Autodesk Inventor part; units mm, degrees
(part 2 of 2)
  spline S148 degree 2 poles (-17.7815, 46.7577) (-17.6758, 46.9585) (-17.3312, 47.2573) (-17.0296, 47.3658) knots 0 0 0 1 2 2 2
  spline S149 degree 2 poles (-19.8158, 45.9019) (-19.7815, 45.9593) (-19.669, 46.1603) (-19.607, 46.2324) knots 0 0 0 1 2 2 2
  spline S150 degree 2 poles (-19.607, 46.2324) (-19.5238, 46.335) (-19.3477, 46.4796) (-19.1646, 46.5564) knots 0 0 0 1 2 2 2
  spline S151 degree 2 poles (-19.1646, 46.5564) (-19.0155, 46.6189) (-18.6989, 46.6194) (-18.5541, 46.5602) knots 0 0 0 1 2 2 2
  spline S152 degree 2 poles (-18.5541, 46.5602) (-18.4157, 46.5014) (-18.1751, 46.2578) (-18.1071, 46.0957) knots 0 0 0 1 2 2 2
  spline S153 degree 2 poles (-18.1071, 46.0957) (-18.0018, 45.8446) (-18.0645, 45.4) (-18.2518, 45.2014) knots 0 0 0 1 2 2 2
  spline S154 degree 2 poles (-18.2518, 45.2014) (-18.4164, 45.0217) (-18.9413, 44.7185) (-19.2553, 44.5653) knots 0 0 0 1 2 2 2
  line L139 (-19.2553, 44.5653) -> (-19.2224, 44.4868)
  spline S155 degree 2 poles (-19.2224, 44.4868) (-19.1631, 44.3456) (-19.0033, 44.2065) (-18.904, 44.1898) knots 0 0 0 1 2 2 2
  spline S156 degree 2 poles (-18.904, 44.1898) (-18.8047, 44.173) (-18.5666, 44.2359) (-18.4463, 44.2864) knots 0 0 0 1 2 2 2
  spline S157 degree 2 poles (-18.4463, 44.2864) (-18.305, 44.3456) (-17.9583, 44.5895) (-17.8013, 44.7506) knots 0 0 0 1 2 2 2
  line L140 (-17.8013, 44.7506) -> (-17.7778, 44.7605)
  line L141 (-17.7778, 44.7605) -> (-17.6034, 44.3446)
  spline S158 degree 2 poles (-17.6034, 44.3446) (-17.7027, 44.2661) (-18.0909, 44.011) (-18.2975, 43.9243) knots 0 0 0 1 2 2 2
  spline S159 degree 2 poles (-18.2975, 43.9243) (-18.5486, 43.819) (-18.9242, 43.7538) (-19.103, 43.7988) knots 0 0 0 1 2 2 2
  spline S160 degree 2 poles (-19.103, 43.7988) (-19.278, 43.8422) (-19.5416, 44.1038) (-19.637, 44.3314) knots 0 0 0 1 2 2 2
  line L142 (-19.637, 44.3314) -> (-20.3314, 45.9871)
  line L143 (-20.3314, 45.9871) -> (-19.9234, 46.1582)
  line L144 (-19.9234, 46.1582) -> (-19.8158, 45.9019)
  line L145 (-19.6732, 45.5618) -> (-19.3913, 44.8896)
  spline S161 degree 2 poles (-19.3913, 44.8896) (-19.2503, 44.9641) (-18.8269, 45.194) (-18.7059, 45.294) knots 0 0 0 1 2 2 2
  spline S162 degree 2 poles (-18.7059, 45.294) (-18.5645, 45.4117) (-18.4393, 45.7072) (-18.5161, 45.8903) knots 0 0 0 1 2 2 2
  spline S163 degree 2 poles (-18.5161, 45.8903) (-18.6039, 46.0995) (-18.9282, 46.2126) (-19.1531, 46.1183) knots 0 0 0 1 2 2 2
  spline S164 degree 2 poles (-19.1531, 46.1183) (-19.344, 46.0382) (-19.5888, 45.7418) (-19.6732, 45.5618) knots 0 0 0 1 2 2 2
  line L146 (-21.3036, 45.5352) -> (-20.902, 45.7209)
  line L147 (-20.902, 45.7209) -> (-19.3673, 42.4026)
  line L148 (-19.3673, 42.4026) -> (-19.7689, 42.2169)
  line L149 (-19.7689, 42.2169) -> (-21.3036, 45.5352)
  line L150 (-23.4333, 44.4869) -> (-21.7097, 45.3524)
  line L151 (-21.7097, 45.3524) -> (-21.5621, 45.0584)
  line L152 (-21.5621, 45.0584) -> (-21.9207, 42.7137)
  line L153 (-21.9207, 42.7137) -> (-20.7446, 43.3043)
  line L154 (-20.7446, 43.3043) -> (-20.5817, 42.9799)
  line L155 (-20.5817, 42.9799) -> (-22.2317, 42.1513)
  line L156 (-22.2317, 42.1513) -> (-22.373, 42.4326)
  line L157 (-22.373, 42.4326) -> (-22.0119, 44.7849)
  line L158 (-22.0119, 44.7849) -> (-23.2665, 44.1548)
  line L159 (-23.2665, 44.1548) -> (-23.4333, 44.4869)
  spline S165 degree 2 poles (-25.051, 42.0314) (-25.3671, 42.5923) (-25.2091, 43.5831) (-24.7989, 43.8143) knots 0 0 0 1 2 2 2
  spline S166 degree 2 poles (-24.7989, 43.8143) (-24.6136, 43.9187) (-24.2977, 43.9762) (-24.1246, 43.9696) knots 0 0 0 1 2 2 2
  line L160 (-24.1246, 43.9696) -> (-24.1598, 44.0897)
  line L161 (-24.1598, 44.0897) -> (-23.799, 44.293)
  line L162 (-23.799, 44.293) -> (-22.0043, 41.1079)
  line L163 (-22.0043, 41.1079) -> (-22.3898, 40.8907)
  line L164 (-22.3898, 40.8907) -> (-23.0302, 42.0273)
  spline S167 degree 2 poles (-23.0302, 42.0273) (-23.1022, 41.8142) (-23.3433, 41.4505) (-23.5583, 41.3294) knots 0 0 0 1 2 2 2
  spline S168 degree 2 poles (-23.5583, 41.3294) (-23.9462, 41.1108) (-24.7405, 41.4804) (-25.051, 42.0314) knots 0 0 0 1 2 2 2
  spline S169 degree 2 poles (-24.6699, 42.2852) (-24.4387, 41.875) (-23.9497, 41.5907) (-23.6729, 41.7466) knots 0 0 0 1 2 2 2
  spline S170 degree 2 poles (-23.6729, 41.7466) (-23.5173, 41.8343) (-23.2796, 42.1636) (-23.2126, 42.351) knots 0 0 0 1 2 2 2
  line L165 (-23.2126, 42.351) -> (-23.952, 43.6632)
  spline S171 degree 2 poles (-23.952, 43.6632) (-24.1382, 43.6527) (-24.3964, 43.5853) (-24.5299, 43.5101) knots 0 0 0 1 2 2 2
  spline S172 degree 2 poles (-24.5299, 43.5101) (-24.8239, 43.3444) (-24.9247, 42.7374) (-24.6699, 42.2852) knots 0 0 0 1 2 2 2
  line L166 (-27.8316, 41.8771) -> (-27.4582, 42.1144)
  line L167 (-27.4582, 42.1144) -> (-27.303, 41.8703)
  spline S173 degree 2 poles (-27.303, 41.8703) (-27.2266, 42.1307) (-27.0167, 42.4825) (-26.8252, 42.6043) knots 0 0 0 1 2 2 2
  spline S174 degree 2 poles (-26.8252, 42.6043) (-26.6816, 42.6956) (-26.3646, 42.7626) (-26.2058, 42.719) knots 0 0 0 1 2 2 2
  spline S175 degree 2 poles (-26.2058, 42.719) (-26.0447, 42.677) (-25.74, 42.4304) (-25.597, 42.2054) knots 0 0 0 1 2 2 2
  line L168 (-25.597, 42.2054) -> (-24.6825, 40.7668)
  line L169 (-24.6825, 40.7668) -> (-25.0559, 40.5295)
  line L170 (-25.0559, 40.5295) -> (-25.8593, 41.7933)
  spline S176 degree 2 poles (-25.8593, 41.7933) (-25.9719, 41.9704) (-26.1458, 42.1858) (-26.2461, 42.2431) knots 0 0 0 1 2 2 2
  spline S177 degree 2 poles (-26.2461, 42.2431) (-26.3463, 42.3004) (-26.5521, 42.2804) (-26.6981, 42.1876) knots 0 0 0 1 2 2 2
  spline S178 degree 2 poles (-26.6981, 42.1876) (-26.8346, 42.1009) (-27.0444, 41.749) (-27.1022, 41.5543) knots 0 0 0 1 2 2 2
  line L171 (-27.1022, 41.5543) -> (-26.0492, 39.898)
  line L172 (-26.0492, 39.898) -> (-26.4226, 39.6606)
  line L173 (-26.4226, 39.6606) -> (-27.8316, 41.8771)
  line L174 (-28.2667, 38.9506) -> (-28.2481, 38.9636)
  spline S179 degree 2 poles (-28.2481, 38.9636) (-28.1981, 38.9812) (-28.1042, 39.0399) (-28.0414, 39.0838) knots 0 0 0 1 2 2 2
  spline S180 degree 2 poles (-28.0414, 39.0838) (-27.895, 39.1862) (-27.6962, 39.5156) (-27.6537, 39.7321) knots 0 0 0 1 2 2 2
  line L175 (-27.6537, 39.7321) -> (-28.7216, 41.2593)
  line L176 (-28.7216, 41.2593) -> (-28.359, 41.5128)
  line L177 (-28.359, 41.5128) -> (-26.8539, 39.3604)
  line L178 (-26.8539, 39.3604) -> (-27.2165, 39.1069)
  line L179 (-27.2165, 39.1069) -> (-27.4408, 39.4276)
  spline S181 degree 2 poles (-27.4408, 39.4276) (-27.5149, 39.1128) (-27.7093, 38.7623) (-27.8488, 38.6648) knots 0 0 0 1 2 2 2
  spline S182 degree 2 poles (-27.8488, 38.6648) (-27.9046, 38.6258) (-27.9636, 38.5914) (-28.0034, 38.574) knots 0 0 0 1 2 2 2
  line L180 (-28.0034, 38.574) -> (-28.2667, 38.9506)
  spline S183 degree 2 poles (-30.1088, 40.7913) (-30.1569, 40.7794) (-30.3322, 40.7237) (-30.4355, 40.6767) knots 0 0 0 1 2 2 2
  spline S184 degree 2 poles (-30.4355, 40.6767) (-30.5513, 40.6272) (-30.7381, 40.5306) (-30.8349, 40.4564) knots 0 0 0 1 2 2 2
  spline S185 degree 2 poles (-30.8349, 40.4564) (-30.9969, 40.3321) (-31.1565, 40.0741) (-31.1609, 39.9492) knots 0 0 0 1 2 2 2
  spline S186 degree 2 poles (-31.1609, 39.9492) (-31.163, 39.8261) (-31.0567, 39.5895) (-30.9584, 39.4612) knots 0 0 0 1 2 2 2
  line L181 (-30.9584, 39.4612) -> (-30.8186, 39.2788)
  spline S187 degree 2 poles (-30.8186, 39.2788) (-30.7717, 39.5114) (-30.589, 39.8372) (-30.3842, 39.9942) knots 0 0 0 1 2 2 2
  spline S188 degree 2 poles (-30.3842, 39.9942) (-30.0285, 40.2668) (-29.202, 40.0604) (-28.8207, 39.5629) knots 0 0 0 1 2 2 2
  spline S189 degree 2 poles (-28.8207, 39.5629) (-28.6223, 39.304) (-28.4615, 38.7911) (-28.4744, 38.5562) knots 0 0 0 1 2 2 2
  spline S190 degree 2 poles (-28.4744, 38.5562) (-28.4897, 38.3336) (-28.6994, 37.9406) (-28.8705, 37.8094) knots 0 0 0 1 2 2 2
  spline S191 degree 2 poles (-28.8705, 37.8094) (-29.0326, 37.6852) (-29.3277, 37.5806) (-29.5005, 37.5589) knots 0 0 0 1 2 2 2
  line L182 (-29.5005, 37.5589) -> (-29.4534, 37.4556)
  line L183 (-29.4534, 37.4556) -> (-29.7844, 37.202)
  line L184 (-29.7844, 37.202) -> (-31.1991, 39.048)
  spline S192 degree 2 poles (-31.1991, 39.048) (-31.6063, 39.5792) (-31.5244, 40.4282) (-31.0494, 40.7922) knots 0 0 0 1 2 2 2
  spline S193 degree 2 poles (-31.0494, 40.7922) (-30.8963, 40.9096) (-30.5387, 41.105) (-30.3703, 41.1698) knots 0 0 0 1 2 2 2
  line L185 (-30.3703, 41.1698) -> (-30.0908, 40.8051)
  line L186 (-30.0908, 40.8051) -> (-30.1088, 40.7913)
  line L187 (-30.5978, 38.9907) -> (-29.7196, 37.8448)
  spline S194 degree 2 poles (-29.7196, 37.8448) (-29.5407, 37.8819) (-29.2787, 37.9969) (-29.1684, 38.0815) knots 0 0 0 1 2 2 2
  spline S195 degree 2 poles (-29.1684, 38.0815) (-28.9027, 38.2851) (-28.8968, 38.9114) (-29.178, 39.2784) knots 0 0 0 1 2 2 2
  spline S196 degree 2 poles (-29.178, 39.2784) (-29.4437, 39.625) (-29.9534, 39.8098) (-30.2145, 39.6096) knots 0 0 0 1 2 2 2
  spline S197 degree 2 poles (-30.2145, 39.6096) (-30.3518, 39.5044) (-30.5572, 39.1755) (-30.5978, 38.9907) knots 0 0 0 1 2 2 2
  constraints: 1 centre point, 1 coincident, 1 other
extrude "Extrusion3" add sketch "Skizze3" along normal blind 1 contours S0 S1 L0 L1 L2 L3 L4 S2 S3 | S8 S9 S10 S11 S12 S13 L8 S14 S15 S16 L9 L10 S17 S18 S19 L11 L12 L13 | L15 S24 S25 L16 L17 L18 L19 L20 S26 S27 L21 | L22 L23 L24 L25 | L26 L27 L28 L29 | S28 L30 L31 S29 S30 S31 S32 S33 S34 S35 S36 S37 L32 L33 S38 S39 S40 S41 S42 S43 S44 | L34 L35 L36 L37 L38 L39 | S45 S46 S47 S48 | L40 L41 S53 S54 S55 S56 S57 S58 S59 L42 L43 L44 | L46 S64 S65 L47 L48 L49 L50 L51 S66 S67 L52 | S68 S69 S70 S71 | L53 L54 S76 S77 S78 L55 L56 L57 L58 L59 S79 S80 L60 | S81 S82 L61 L62 L63 S83 S84 S85 S86 L64 L65 L66 S87 S88 | L67 L68 S89 S90 S91 L69 L70 L71 L72 L73 S92 S93 L74 | L75 L76 L77 L78 | L79 L80 L81 L82 | L83 L84 L85 L86 L87 L88 L89 | S94 S95 S96 S97 L90 L91 S98 S99 S100 L92 L93 S101 S102 | L95 S107 S108 L96 L97 L98 L99 L100 S109 S110 L101 | S111 L102 L103 S112 S113 S114 S115 S116 S117 S118 S119 S120 L104 L105 S121 S122 S123 S124 S125 S126 S127 | L106 L107 L108 L109 | L110 L111 L112 L113 | S128 L114 L115 L116 L117 L118 L119 L120 L121 L122 L131 L130 L123 L124 S129 S130 S131 L125 L126 S132 | L130 L131 L122 | L122 L131 L132 L133 L134 L127 L128 L129 L130 | S133 L135 L136 S134 S135 S136 S137 S138 S139 S140 S141 L137 L138 S142 S143 S144 S145 S146 S147 S148 | S149 S150 S151 S152 S153 S154 L139 S155 S156 S157 L140 L141 S158 S159 S160 L142 L143 L144 | L146 L147 L148 L149 | L150 L151 L152 L153 L154 L155 L156 L157 L158 L159 | S165 S166 L160 L161 L162 L163 L164 S167 S168 | L166 L167 S173 S174 S175 L168 L169 L170 S176 S177 S178 L171 L172 L173 | L174 S179 S180 L175 L176 L177 L178 L179 S181 S182 L180 | S183 S184 S185 S186 L181 S187 S188 S189 S190 S191 L182 L183 L184 S192 S193 L185 L186
ref_plane "Arbeitsebene1" through (0, 0, 0) normal (0, 0, 1) x (1, 0, 0)
